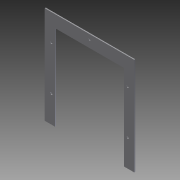
# Autodesk Inventor part: middle-top spacer plate
Saved by Autodesk Inventor 2011 SP1 (Build 150282100, 282)
## iProperties
Created: 2012-01-20
Part Number: middle-top spacer plate
Document SubType Name: Modeling
Designer: Christopher
Density: 1 g/cm^3
Author: Christopher
Autodesk Inventor part; units mm, degrees
ref_plane "YZ Plane" through (0, 0, 0) normal (1, 0, 0) x (0, 1, 0)
ref_plane "XZ Plane" through (0, 0, 0) normal (0, 1, 0) x (-1, 0, 0)
ref_plane "XY Plane" through (0, 0, 0) normal (0, 0, 1) x (1, 0, 0)
sketch "Sketch1" plane through (0, 0, 0) normal (0, 0, 1) x (1, 0, 0)
  line L0 (279.4, 0) -> (279.4, 304.8)
  line L1 (279.4, 304.8) -> (0, 304.8)
  line L2 (0, 304.8) -> (0, 0)
  line L3 (31.75, 0) -> (31.75, 266.7)
  line L4 (31.75, 266.7) -> (247.65, 266.7)
  line L5 (247.65, 266.7) -> (247.65, 0)
  line L6 (247.65, 0) -> (279.4, 0)
  line L7 (31.75, 0) -> (0, 0)
  point P0 (139.7, 152.4)
  point P1 (139.7, 289.941)
  point P2 (20.586, 221.1705)
  point P3 (20.586, 83.6295)
  point P4 (139.7, 14.859)
  point P5 (258.814, 83.6295)
  point P6 (258.814, 221.1705)
  dimension "d0" = 279.4
  dimension "d1" = 304.8
  dimension "d2" = 139.7
  dimension "d3" = 152.4
  dimension "d4" = 137.541
  dimension "d7" = 360
  dimension "d9" = 31.75
  dimension "d10" = 31.75
  dimension "d11" = 38.1
  constraints: 16 end point, 2 parallel, 2 perpendicular, 1 collinear, 7 other
  measures "d0" distance of L1.end L0.end
  measures "d1" distance of L0.end L0.start
  measures "d2" distance from line of L2 point (139.7, 152.4)
  measures "d3" distance from line of L1 point (139.7, 152.4)
  measures "d4" distance of point (139.7, 289.941) point (139.7, 152.4)
  measures "d9" distance between parallel lines of L0 L5
  measures "d10" distance between parallel lines of L2 L3
  measures "d11" distance between parallel lines of L1 L4
extrude "Extrusion1" add sketch "Sketch1" against normal blind 3.175
hole "Hole1" at (139.7, 152.4, 0) at (139.7, 289.941, 0) at (20.586, 221.1705, 0) at (20.586, 83.6295, 0) at (139.7, 14.859, 0) at (258.814, 83.6295, 0) at (258.814, 221.1705, 0) direction (0, 0, -1) diameter 6.35 depth 25.4 tip angle 118
body "Solid1"
